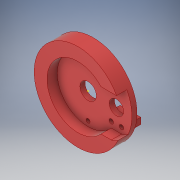
# Autodesk Inventor part: joint2_rotate_mec
Saved by Autodesk Inventor 2019 (Build 230136000, 136)
## iProperties
Created: 2019-12-26
Part Number: joint2_rotate_mec
Material: Пластик АБС
Document SubType Name: Modeling
Designer: Петров Иван
Density: 1.06 g/cm^3
Appearance: Гладкий — красный
Author: Петров Иван
Autodesk Inventor part; units mm, degrees
ref_plane "YZ Plane" through (0, 0, 0) normal (1, 0, 0) x (0, 1, 0)
ref_plane "XZ Plane" through (0, 0, 0) normal (0, 1, 0) x (-1, 0, 0)
ref_plane "XY Plane" through (0, 0, 0) normal (0, 0, 1) x (1, 0, 0)
sketch "Эскиз2" plane through (0, 0, 0) normal (0, 0, 1) x (1, 0, 0)
  circle A0 centre (0, 0) radius 42.5
  dimension "d0" = 85
  constraints: 1 centre point, 1 coincident
  measures "d0" diameter of A0
extrude "Выдавливание1" add sketch "Эскиз2" along normal blind 5
sketch "Эскиз3" plane through (0, 0, 5) normal (0, 0, 1) x (1, 0, 0)
  circle A0 centre (27.5, 0) radius 7
  arc A1 (22.4345, 19.9171) -> (22.4345, -19.9171) centre (0, 0) ccw
  line L0 (32.5655, -19.9171) -> (22.4345, -19.9171)
  arc A2 (32.5655, -19.9171) -> (38.9118, -17.0915) centre (27.5, 0) ccw
  arc A3 (38.9118, -17.0915) -> (37.5441, 19.9171) centre (0, 0) ccw
  line L1 (22.4345, 19.9171) -> (37.5441, 19.9171)
  circle A4 centre (32.45, -14.15) radius 2.15
  circle A5 centre (0, 0) radius 8
  circle A6 centre (22.55, -14.15) radius 2.15
  arc A7 (32.5655, -19.9171) -> (38.9118, -17.0915) centre (27.5, 0) ccw
  line L2 (32.5655, -19.9171) -> (22.4345, -19.9171)
  arc A8 (22.4345, 19.9171) -> (22.4345, -19.9171) centre (0, 0) ccw
  line L3 (22.4345, 19.9171) -> (37.5441, 19.9171)
  arc A9 (37.5441, 19.9171) -> (38.9118, -17.0915) centre (0, 0) ccw
  point P0 (0, -36.1)
  constraints: 12 point on circle, 10 centre point, 8 end point
extrude "Выдавливание2" add sketch "Эскиз3" along normal blind 10 contours A1 L0 A2 A9 L1
sketch "Эскиз4" plane through (0, 0, 5) normal (0, 0, 1) x (1, 0, 0)
  circle A0 centre (27.5, 0) radius 7
  arc A1 (22.4345, 19.9171) -> (22.4345, -19.9171) centre (0, 0) ccw
  line L0 (32.5655, -19.9171) -> (22.4345, -19.9171)
  arc A2 (32.5655, -19.9171) -> (38.9118, -17.0915) centre (27.5, 0) ccw
  arc A3 (38.9118, -17.0915) -> (37.5441, 19.9171) centre (0, 0) ccw
  line L1 (22.4345, 19.9171) -> (37.5441, 19.9171)
  circle A4 centre (32.45, -14.15) radius 2.15
  circle A5 centre (0, 0) radius 8
  circle A6 centre (22.55, -14.15) radius 2.15
  arc A7 (32.5655, -19.9171) -> (38.9118, -17.0915) centre (27.5, 0) ccw
  line L2 (32.5655, -19.9171) -> (22.4345, -19.9171)
  arc A8 (22.4345, 19.9171) -> (22.4345, -19.9171) centre (0, 0) ccw
  line L3 (22.4345, 19.9171) -> (37.5441, 19.9171)
  arc A9 (37.5441, 19.9171) -> (38.9118, -17.0915) centre (0, 0) ccw
  point P0 (0, -36.1)
  constraints: 12 point on circle, 10 centre point, 8 end point
extrude "Выдавливание3" cut sketch "Эскиз4" against normal blind 10 contours A0 | A4 | A5 | A6
sketch "Эскиз5" plane through (-19.7699, -0.8287, 0) normal (0, 0, -1) x (-1, 0, 0)
  line L0 (-37.2699, -9.1713) -> (-57.2699, -9.1713)
  line L1 (-57.2699, -9.1713) -> (-57.2699, -15.1713)
  arc A0 (-57.2699, -15.1713) -> (-56.2699, -16.1713) centre (-56.2699, -15.1713) ccw
  line L2 (-56.2699, -16.1713) -> (-53.4199, -16.1713)
  arc A1 (-51.0199, -15.1052) -> (-53.4199, -15.1052) centre (-52.2199, -13.3213) ccw
  line L3 (-51.0199, -16.1713) -> (-43.5199, -16.1713)
  arc A2 (-41.1199, -15.1052) -> (-43.5199, -15.1052) centre (-42.3199, -13.3213) ccw
  line L4 (-41.1199, -16.1713) -> (-38.2699, -16.1713)
  arc A3 (-38.2699, -16.1713) -> (-37.2699, -15.1713) centre (-38.2699, -15.1713) ccw
  line L5 (-37.2699, -15.1713) -> (-37.2699, -9.1713)
  line L6 (-43.5199, 38.5287) -> (-43.5199, 37.4627)
  line L7 (-51.0199, 38.5287) -> (-43.5199, 38.5287)
  line L8 (-51.0199, 37.4627) -> (-51.0199, 38.5287)
  arc A4 (-53.4199, 37.4627) -> (-51.0199, 37.4627) centre (-52.2199, 35.6787) ccw
  line L9 (-53.4199, 38.5287) -> (-53.4199, 37.4627)
  line L10 (-56.2699, 38.5287) -> (-53.4199, 38.5287)
  arc A5 (-56.2699, 38.5287) -> (-57.2699, 37.5287) centre (-56.2699, 37.5287) ccw
  line L11 (-57.2699, 31.5287) -> (-57.2699, 37.5287)
  line L12 (-37.2699, 31.5287) -> (-57.2699, 31.5287)
  line L13 (-37.2699, 37.5287) -> (-37.2699, 31.5287)
  arc A6 (-37.2699, 37.5287) -> (-38.2699, 38.5287) centre (-38.2699, 37.5287) ccw
  line L14 (-41.1199, 38.5287) -> (-38.2699, 38.5287)
  line L15 (-41.1199, 37.4627) -> (-41.1199, 38.5287)
  arc A7 (-43.5199, 37.4627) -> (-41.1199, 37.4627) centre (-42.3199, 35.6787) ccw
  line L16 (-57.2699, -9.1713) -> (-57.2699, 31.5287)
  line L17 (-37.2699, 31.5287) -> (-37.2699, -9.1713)
  line L18 (-37.2699, -9.1713) -> (-57.2699, -9.1713)
  circle A8 centre (-47.2699, 0.8287) radius 1.25
  circle A9 centre (-47.2699, 0.8287) radius 3.4957
  circle A10 centre (-47.2699, 0.8287) radius 2.6787
  circle A11 centre (-47.2699, 0.8287) radius 5.4
  line L19 (-37.2699, -14.1713) -> (-37.2699, 15.8287)
  line L20 (-37.2699, 0.8287) -> (-47.2699, 0.8287)
  circle A12 centre (-52.2199, -13.3213) radius 2.15
  circle A13 centre (-42.3199, -13.3213) radius 2.15
  line L21 (-53.4199, -16.1713) -> (-51.0199, -16.1713)
  line L22 (-43.5199, -16.1713) -> (-40.9117, -16.1713)
  circle A14 centre (-52.2199, -13.3213) radius 2.15 projected
  point P0 (0, -36.1)
  point P1 (0, -36.1)
  point P2 (-37.2699, 11.1787)
  dimension "d7" = 10
  constraints: 46 end point, 16 point on circle, 14 centre point, 2 coincident, 2 concentric, 2 horizontal, 1 midpoint, 1 point on line
  measures "d7" distance of L20.start L20.end
extrude "Выдавливание4" add sketch "Эскиз5" along normal blind 8.6 contours L5 A3 L4 L22 L3 L21 L2 A0 L1 L0
sketch "Эскиз6" plane through (0, 0, 5) normal (0, 0, 1) x (1, 0, 0)
  circle A0 centre (0, 25) radius 1.9
  circle A1 centre (0, -25) radius 1.9
  circle A2 centre (0, 0) radius 8
  line L0 (-17.5, -36.1) -> (17.5, -36.1)
  line L1 (17.5, -36.1) -> (17.5, 36.1)
  line L2 (17.5, 36.1) -> (-17.5, 36.1)
  line L3 (-17.5, 36.1) -> (-17.5, -36.1)
  point P0 (0, -36.1)
  constraints: 8 end point, 3 centre point
extrude "Выдавливание5" cut sketch "Эскиз6" against normal blind 10 contours A0 | A1
sketch "Эскиз7" plane through (0, 0, 5) normal (0, 0, 1) x (1, 0, 0)
  point P0 (0, 0)
